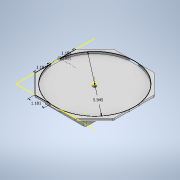
# Autodesk Inventor part: 6in-wafer-adapter-for-hs
Saved by Autodesk Inventor 2020 (Build 240168000, 168)
## iProperties
Created: 2023-06-09
Part Number: 6in-wafer-adapter-for-hs
Material: Generic
Document SubType Name: Modeling
Designer: Beaucage
Density: 1 g/cm^3
Appearance: Default
Author: Beaucage
Autodesk Inventor part; units mm, degrees
ref_plane "YZ Plane" through (0, 0, 0) normal (1, 0, 0) x (0, 1, 0)
ref_plane "XZ Plane" through (0, 0, 0) normal (0, 1, 0) x (-1, 0, 0)
ref_plane "XY Plane" through (0, 0, 0) normal (0, 0, 1) x (1, 0, 0)
sketch "Sketch1" plane through (0, 0, 0) normal (0, 1, 0) x (-1, 0, 0)
  line L0 (0, 0) -> (78, 0)
  line L1 (78, 0) -> (78, -114)
  line L2 (78, -114) -> (0, -114)
  line L3 (0, -114) -> (0, 0)
  dimension "d0" = 78
  dimension "d1" = 114
  constraints: 8 end point, 2 parallel, 1 horizontal, 1 perpendicular
  measures "d0" distance of L1.end L2.end
  measures "d1" distance of L0.end L1.end
extrude "Extrusion1" add sketch "Sketch1" along normal blind 17.5
sketch "Sketch2" plane through (0, 17.5, 0) normal (0, 1, 0) x (1, 0, 0)
  line L0 (-78, 114) -> (-78, 0) projected
  point P0 (0, 0)
  point P1 (-78, 57)
  point P2 (-39, 57)
  constraints: 1 midpoint
hole "Hole1" at (-39, 17.5, -57) direction (0, -1, 0) diameter 6 depth 15.75 tip angle 118
hole "Hole2" at (-39, 17.5, -57) direction (0, -1, 0) diameter 3.5 end through all
sketch "Sketch3" plane through (0, 17.5, 0) normal (0, 1, 0) x (1, 0, 0)
  line L0 (-114, -18) -> (36, -18)
  line L1 (36, -18) -> (36, 132)
  line L2 (36, 132) -> (-114, 132)
  line L3 (-114, 132) -> (-114, -18)
  circle A0 centre (-39, 57) radius 3 projected
  line L4 (-114, -18) -> (36, 132) construction
  line L5 (36, -18) -> (-114, 132) construction
  point P0 (0, 0)
  dimension "d18" = 150
  dimension "d19" = 150
  constraints: 12 end point, 2 midpoint, 2 parallel, 1 horizontal, 1 perpendicular
  measures "d18" distance of L2.end L1.end
  measures "d19" distance of L1.end L0.end
extrude "Extrusion2" add sketch "Sketch3" along normal blind 6
sketch "Sketch4" plane through (0, 23.5, 0) normal (0, 1, 0) x (1, 0, 0)
  circle A0 centre (-39, 57) radius 3 projected
  circle A1 centre (-39, 57) radius 75.5
  line L0 (-114, 132) -> (-114, -18) projected
  line L1 (-114, 48.3253) -> (-114, 18.3253)
  line L2 (-114, 65.6747) -> (-114, 95.6747)
  line L3 (-114, 65.6747) -> (-84, 65.6747) construction
  line L4 (-114, -18) -> (36, -18) projected
  line L5 (-47.6747, -18) -> (-77.6747, -18)
  line L6 (-77.6747, -18) -> (-114, 18.3253)
  point P0 (0, 0)
  dimension "d22" = 151
  dimension "d25" = 30
  dimension "d26" = 30
  dimension "d27" = 90
  dimension "d28" = 30
  constraints: 10 end point, 5 point on line, 3 point on circle, 1 centre point, 1 coincident, 1 collinear, 1 horizontal, 1 perpendicular
  measures "d22" diameter of A1
  measures "d25" distance of L1.start L1.end
  measures "d26" distance of L2.start L2.end
  measures "d27" angle of L3 L2
  measures "d28" distance of L5.start L5.end
extrude "Extrusion3" cut sketch "Sketch4" against normal blind 4 contours A1 L4 L0 | L0 A1 | A1 L4
extrude "Extrusion4" cut sketch "Sketch4" against normal blind 6 contours L6 L4 L0
pattern_circular "Circular Pattern1" count 4 over 360 about axis through (-39, 23.5, -57) along (0, 1, 0) of "Extrusion4"
fillet "Fillet1" radius 3.175 20 edges at (17.8373, 17.5, -0.1627) (36, 17.5, -57) (17.8373, 17.5, -113.8373) (-39, 17.5, -132) (-95.8373, 17.5, -113.8373) (-114, 17.5, -57) (-95.8373, 17.5, -0.1627) (-39, 17.5, 18) (36, 20.5, -18.3253) (-0.3253, 20.5, 18) (36, 20.5, -95.6747) (-0.3253, 20.5, -132) (-77.6747, 20.5, -132) (-114, 20.5, -95.6747) (-114, 20.5, -18.3253) (-77.6747, 20.5, 18) (-78, 8.75, 0) (0, 8.75, 0) (-78, 8.75, -114) (0, 8.75, -114)
body "Solid1"
